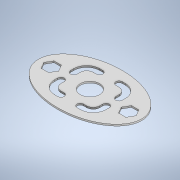
# Autodesk Inventor part: VentCover
Saved by Autodesk Inventor 2022.2 (Build 262287030, 287C)
## iProperties
Created: 2023-04-24
Part Number: VentCover
Material: Generic
Document SubType Name: Modeling
Designer: jak27277
Density: 1 g/cm^3
Appearance: Default
Author: jak27277
Autodesk Inventor part; units mm, degrees
ref_plane "YZ Plane" through (0, 0, 0) normal (1, 0, 0) x (0, 1, 0)
ref_plane "XZ Plane" through (0, 0, 0) normal (0, 1, 0) x (-1, 0, 0)
ref_plane "XY Plane" through (0, 0, 0) normal (0, 0, 1) x (1, 0, 0)
sketch "Sketch1" plane through (0, 0, 0) normal (0, 1, 0) x (-1, 0, 0)
  ellipse E0 centre (0, 0) end of major axis (-101.6, 0) minor radius 63.5
  circle A0 centre (0, 0) radius 19.05
  arc A1 (-25.4, 38.1) -> (-44.45, 19.05) centre (-25.4, 19.05) ccw construction
  line L0 (-44.45, 19.05) -> (-44.45, 12.7) construction
  line L1 (-25.4, 38.1) -> (-19.05, 38.1) construction
  line L2 (-38.1, 12.7) -> (-38.1, 19.05)
  arc A2 (-25.4, 31.75) -> (-38.1, 19.05) centre (-25.4, 19.05) ccw
  line L3 (-25.4, 31.75) -> (-19.05, 31.75)
  arc A3 (-19.05, 31.75) -> (-19.05, 44.45) centre (-19.05, 38.1) ccw
  arc A4 (-50.8, 12.7) -> (-38.1, 12.7) centre (-44.45, 12.7) ccw
  line L4 (-50.8, 12.7) -> (-50.8, 19.05)
  line L5 (-19.05, 44.45) -> (-25.4, 44.45)
  arc A5 (-25.4, 44.45) -> (-50.8, 19.05) centre (-25.4, 19.05) ccw
  line L6 (0, 0) -> (0, -63.5) construction
  line L7 (0, 0) -> (-101.6, 0) construction
  line L8 (38.1, 12.7) -> (38.1, 19.05)
  arc A6 (38.1, 19.05) -> (25.4, 31.75) centre (25.4, 19.05) ccw
  line L9 (25.4, 31.75) -> (19.05, 31.75)
  arc A7 (19.05, 44.45) -> (19.05, 31.75) centre (19.05, 38.1) ccw
  arc A8 (38.1, 12.7) -> (50.8, 12.7) centre (44.45, 12.7) ccw
  line L10 (50.8, 12.7) -> (50.8, 19.05)
  line L11 (19.05, 44.45) -> (25.4, 44.45)
  arc A9 (50.8, 19.05) -> (25.4, 44.45) centre (25.4, 19.05) ccw
  line L12 (0, 0) -> (101.6, 0) construction
  arc A10 (-44.45, -19.05) -> (-25.4, -38.1) centre (-25.4, -19.05) ccw construction
  line L13 (-44.45, -19.05) -> (-44.45, -12.7) construction
  line L14 (-38.1, -12.7) -> (-38.1, -19.05)
  arc A11 (-38.1, -19.05) -> (-25.4, -31.75) centre (-25.4, -19.05) ccw
  line L15 (-25.4, -31.75) -> (-19.05, -31.75)
  arc A12 (-19.05, -44.45) -> (-19.05, -31.75) centre (-19.05, -38.1) ccw
  arc A13 (-38.1, -12.7) -> (-50.8, -12.7) centre (-44.45, -12.7) ccw
  line L16 (-50.8, -12.7) -> (-50.8, -19.05)
  line L17 (-19.05, -44.45) -> (-25.4, -44.45)
  arc A14 (-50.8, -19.05) -> (-25.4, -44.45) centre (-25.4, -19.05) ccw
  line L18 (0, 0) -> (0, 63.5) construction
  arc A15 (25.4, -44.45) -> (50.8, -19.05) centre (25.4, -19.05) ccw
  line L19 (50.8, -12.7) -> (50.8, -19.05)
  arc A16 (50.8, -12.7) -> (38.1, -12.7) centre (44.45, -12.7) ccw
  line L20 (38.1, -12.7) -> (38.1, -19.05)
  arc A17 (25.4, -31.75) -> (38.1, -19.05) centre (25.4, -19.05) ccw
  line L21 (25.4, -31.75) -> (19.05, -31.75)
  arc A18 (19.05, -31.75) -> (19.05, -44.45) centre (19.05, -38.1) ccw
  line L22 (19.05, -44.45) -> (25.4, -44.45)
  line L23 (-68.8677, -12.7) -> (-83.5323, -12.7)
  line L24 (-83.5323, -12.7) -> (-90.8647, 0)
  line L25 (-90.8647, 0) -> (-83.5323, 12.7)
  line L26 (-83.5323, 12.7) -> (-68.8677, 12.7)
  line L27 (-68.8677, 12.7) -> (-61.5353, 0)
  line L28 (-61.5353, 0) -> (-68.8677, -12.7)
  line L29 (0, 0) -> (101.6, 0) construction
  line L30 (68.8677, -12.7) -> (83.5323, -12.7)
  line L31 (83.5323, -12.7) -> (90.8647, 0)
  line L32 (90.8647, 0) -> (83.5323, 12.7)
  line L33 (83.5323, 12.7) -> (68.8677, 12.7)
  line L34 (68.8677, 12.7) -> (61.5353, 0)
  line L35 (61.5353, 0) -> (68.8677, -12.7)
  point P0 (-76.2, 0)
  point P1 (76.2, 0)
  dimension "d0" = 101.6
  dimension "d1" = 63.5
  dimension "d5" = 25.4
  dimension "d6" = 19.05
  dimension "d7" = 19.05
  dimension "d8" = 6.35
  dimension "d9" = 6.35
  dimension "d10" = 38.1
  dimension "d11" = 76.2
  dimension "d12" = 25.4
  constraints: 72 end point, 48 symmetric about line, 36 point on circle, 19 centre point, 9 coincident, 6 tangent, 4 horizontal, 3 vertical, 2 point on line, 1 equal radius, 1 perpendicular, 32 other
  measures "d5" horizontal distance of A1.centre point (0, 0)
  measures "d6" vertical distance of point (0, 0) A1.centre
  measures "d7" radius of A1
  measures "d8" distance of L0.start L0.end
  measures "d9" radius of A4
  measures "d10" diameter of A0
  measures "d11" distance of point (-76.2, 0) point (0, 0)
  measures "d12" distance between parallel lines of L26 L23
extrude "Extrusion1" add sketch "Sketch1" along normal blind 3.175
body "Solid1"
